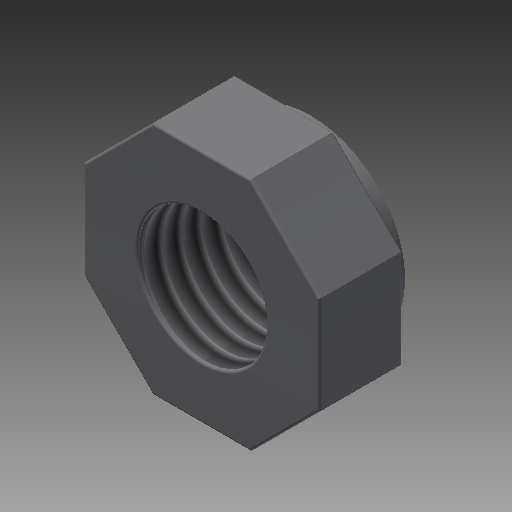
# Autodesk Inventor part: 202-11
Saved by Autodesk Inventor 2019 (Build 230136000, 136)
## iProperties
Company: Autodesk Inc.
Created: 2007-11-01
Part Number: 202-11
Document SubType Name: Modeling
Designer: Autodesk Inc.
Density: 8 g/cm^3
Mass: 11.7295 g
Surface Area: 11.3549 cm^2
Volume: 1.46619 cm^3
Material: Stainless Steel
Description: N34 NUT M12
Appearance: Light Gray
Component Category: Fasteners
Author: Inventor
Autodesk Inventor part; units mm, degrees
ref_plane "YZ Plane" through (0, 0, 0) normal (1, 0, 0) x (0, 1, 0)
ref_plane "XZ Plane" through (0, 0, 0) normal (0, 1, 0) x (-1, 0, 0)
ref_plane "XY Plane" through (0, 0, 0) normal (0, 0, 1) x (1, 0, 0)
sketch "Sketch1" plane through (0, 0, 0) normal (0, 0, 1) x (1, 0, 0)
  line L0 (-12.8051, 0) -> (12.8051, 0) projected
  line L1 (9.1465, -3.7886) -> (3.7886, -9.1465)
  line L2 (3.7886, -9.1465) -> (-3.7886, -9.1465)
  line L3 (-3.7886, -9.1465) -> (-9.1465, -3.7886)
  line L4 (-9.1465, -3.7886) -> (-9.1465, 3.7886)
  line L5 (-9.1465, 3.7886) -> (-3.7886, 9.1465)
  line L6 (-3.7886, 9.1465) -> (3.7886, 9.1465)
  line L7 (3.7886, 9.1465) -> (9.1465, 3.7886)
  line L8 (9.1465, 3.7886) -> (9.1465, -3.7886)
  circle A0 centre (0, 0) radius 5
  point P0 (9.1465, 0)
  dimension "d0" = 18.293
  dimension "d1" = 10
  constraints: 16 end point, 2 coincident, 1 centre point, 1 midpoint, 1 point on line, 17 other
  measures "d0" distance between parallel lines of L8 L4
  measures "d1" diameter of A0
extrude "Extrusion1" add sketch "Sketch1" against normal blind 6.48 contours L4 L5 L6 L7 L8 L0 A0 | L0 A0 L8 L1 L2 L3 L4
sketch "Sketch2" plane through (0, 0, -6.48) normal (0, 0, -1) x (-1, 0, 0)
  circle A0 centre (0, 0) radius 5 projected
  circle A1 centre (0, 0) radius 7.325
  dimension "d4" = 14.65
  constraints: 1 centre point, 1 coincident
  measures "d4" diameter of A1
extrude "Extrusion2" add sketch "Sketch2" along normal blind 2
fillet "Fillet1" radius 0.2 17 edges at (0, -9.1465, 0) (-6.4676, -6.4676, 0) (6.4676, -6.4676, 0) (9.1465, 0, 0) (6.4676, 6.4676, 0) (0, 9.1465, 0) (-6.4676, 6.4676, 0) (-9.1465, 0, 0) (9.1465, 0, -6.48) (6.4676, -6.4676, -6.48) (0, -9.1465, -6.48) (-6.4676, -6.4676, -6.48) (-9.1465, 0, -6.48) (-6.4676, 6.4676, -6.48) (0, 9.1465, -6.48) (6.4676, 6.4676, -6.48) (-5, 0, 0)
thread "Thread1" size "M10x1.5" class "6H" standard "ANSI Metric M Profile" full length
body "Solid1"
